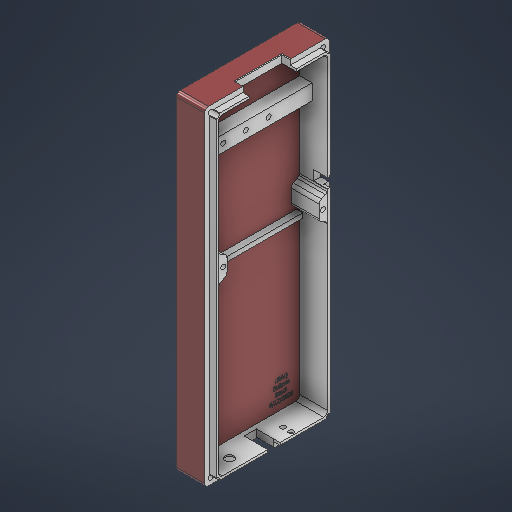
# Autodesk Inventor part: cDAQ_Bottom_Box3
Saved by Autodesk Inventor 2027 (Build 310192000, 192)
## iProperties
Created: 2026-05-08
Part Number: cDAQ_Bottom_Box3
Material: Generic
Document SubType Name: Modeling
Designer: giese
Density: 1 g/cm^3
Appearance: Default
Author: giese
Autodesk Inventor part; units mm, degrees
(part 1 of 2)
ref_plane "YZ Plane" through (0, 0, 0) normal (1, 0, 0) x (0, 1, 0)
ref_plane "XZ Plane" through (0, 0, 0) normal (0, 1, 0) x (-1, 0, 0)
ref_plane "XY Plane" through (0, 0, 0) normal (0, 0, 1) x (1, 0, 0)
sketch "Sketch1" plane through (0, 0, 0) normal (1, 0, 0) x (0, 1, 0)
  line L0 (37.5698, 53.1667) -> (-230.1462, 53.1667)
  line L1 (-230.1462, 53.1667) -> (-230.1462, -48.4333)
  line L2 (-230.1462, -48.4333) -> (37.5698, -48.4333)
  line L3 (37.5698, -48.4333) -> (37.5698, 53.1667)
  point P0 (0, 0)
  dimension "d0" = 101.6
  dimension "d1" = 267.716
  constraints: 8 end point, 2 parallel, 1 horizontal, 1 perpendicular
  measures "d0" distance of L2.end L0.start
  measures "d1" distance of L1.end L2.end
extrude "Extrusion1" add sketch "Sketch1" along normal blind 22.86
sketch "Sketch2" plane through (22.86, 0, 0) normal (1, 0, 0) x (0, 0, -1)
  line L0 (42.0833, 31.2198) -> (-46.8167, 31.2198)
  line L1 (-46.8167, 31.2198) -> (-46.8167, -223.7962)
  line L2 (-46.8167, -223.7962) -> (42.0833, -223.7962)
  line L3 (42.0833, -223.7962) -> (42.0833, 31.2198)
  line L4 (48.4333, 37.5698) -> (-53.1667, 37.5698) projected
  line L5 (-53.1667, 37.5698) -> (-53.1667, -230.1462) projected
  line L6 (-53.1667, -230.1462) -> (48.4333, -230.1462) projected
  point P0 (0, 0)
  dimension "d4" = 255.016
  dimension "d5" = 88.9
  dimension "d8" = 6.35
  dimension "d21" = 6.35
  dimension "d690" = 6.35
  constraints: 8 end point, 2 parallel, 1 horizontal, 1 perpendicular
  measures "d4" distance of L2.end L0.start
  measures "d5" distance of L0.start L0.end
  measures "d8" distance between parallel lines of L0 L4
  measures "d21" distance between parallel lines of L5 L1
  measures "d690" distance between parallel lines of L6 L2
extrude "Extrusion2" cut sketch "Sketch2" against normal blind 17.78
sketch "Sketch3" plane through (0, 0, 0) normal (-1, 0, 0) x (0, 0, 1)
  circle A0 centre (-6.6909, -2.0542) radius 2
  circle A1 centre (11.8079, -2.0542) radius 2
  circle A2 centre (30.3067, -2.0542) radius 2
  line L0 (-48.4333, -230.1462) -> (-48.4333, 37.5698) projected
  line L1 (-48.4333, 37.5698) -> (53.1667, 37.5698) projected
  line L2 (53.1667, 37.5698) -> (53.1667, -230.1462) projected
  line L3 (46.8167, 31.2198) -> (-42.0833, 31.2198) projected
  point P0 (0, 0)
  point P1 (-0.896, -23.7433)
  point P2 (-45.1848, 27.0137)
  dimension "d9" = 18.4988
  dimension "d10" = 4
  dimension "d11" = 4
  dimension "d12" = 18.4988
  dimension "d13" = 36.9976
  dimension "d18" = 22.86
  dimension "d22" = 4
  dimension "d58" = 39.624
  constraints: 3 centre point
  measures "d9" distance of A0.centre A1.centre
  measures "d10" diameter of A1
  measures "d11" diameter of A2
  measures "d12" distance of A1.centre A2.centre
  measures "d13" distance of A0.centre A2.centre
  measures "d18" distance from line of L2 A2.centre
  measures "d22" diameter of A0
  measures "d58" distance from line of L1 A2.centre
extrude "Extrusion3" cut sketch "Sketch3" against normal blind 5.08
sketch "Sketch5" plane through (0, -230.1462, -48.4333) normal (0, 0, -1) x (-1, 0, 0)
  line L0 (-27.2034, 165.862) -> (-16.51, 165.862)
  line L1 (-16.51, 165.862) -> (-16.51, 173.862)
  line L2 (-16.51, 173.862) -> (-27.2034, 173.862)
  line L3 (-27.2034, 173.862) -> (-27.2034, 165.862)
  line L4 (0, 267.716) -> (-22.86, 267.716) projected
  line L5 (0, 0) -> (0, 267.716) projected
  line L6 (-22.86, 0) -> (-22.86, 267.716) projected
  point P0 (0, 230.1462)
  point P1 (-21.8567, 173.862)
  point P2 (-21.8567, 165.862)
  dimension "d28" = 10.6934
  dimension "d30" = 8
  dimension "d31" = 16.51
  dimension "d34" = 101.854
  dimension "d215" = 4.3434
  constraints: 8 end point, 2 midpoint, 2 parallel, 1 horizontal, 1 perpendicular
  measures "d28" distance between parallel lines of L1 L3
  measures "d30" distance of point (-21.857, 173.862) point (-21.857, 165.862)
  measures "d31" distance between parallel lines of L5 L1
  measures "d34" distance between parallel lines of L4 L0
  measures "d215" distance between parallel lines of L6 L3
extrude "Extrusion4" cut sketch "Sketch5" against normal blind 24.13
sketch "Sketch6" plane through (0, -230.1462, -48.4333) normal (0, -1, 0) x (1, 0, 0)
  line L0 (24.08, 55.136) -> (16.08, 55.136)
  line L1 (16.08, 45.136) -> (24.08, 45.136)
  line L2 (0, 101.6) -> (0, 0) projected
  line L3 (28.36, 53.1359) -> (28.36, 47.136)
  line L4 (24.08, 55.136) -> (28.36, 53.1359)
  line L5 (28.36, 47.136) -> (24.08, 45.136)
  line L6 (0, 0) -> (22.86, 0) projected
  line L7 (22.86, 95.25) -> (22.86, 6.35) projected
  line L8 (22.86, 41.9134) -> (22.86, 37.4697)
  line L9 (16.08, 55.136) -> (8.636, 55.136)
  line L10 (8.636, 55.136) -> (8.636, 45.136)
  line L11 (8.636, 45.136) -> (21.16, 45.136)
  point P0 (0, 48.4333)
  point P1 (20.08, 55.136)
  point P2 (20.08, 45.136)
  point P3 (16.08, 50.136)
  dimension "d39" = 6
  dimension "d48" = 55.136
  dimension "d221" = 0
  dimension "d223" = 2
  dimension "d224" = 2
  dimension "d225" = 5.5
  dimension "d227" = 4.28
  dimension "d672" = 8.636
  constraints: 18 end point, 2 horizontal, 2 midpoint, 2 parallel, 2 point on line, 1 perpendicular, 1 vertical
  measures "d39" distance of L3.start L3.end
  measures "d48" distance between parallel lines of L6 L0
  measures "d221" horizontal distance of L0.start L1.end
  measures "d223" vertical distance of L3.end L1.end
  measures "d224" vertical distance of L0.start L3.start
  measures "d225" distance between parallel lines of L3 L7
  measures "d227" distance from line of L1.end L3
  measures "d672" distance between parallel lines of L2 L10
extrude "Extrusion5" cut sketch "Sketch6" against normal blind 6.35
sketch "Sketch7" plane through (0, 37.5698, 53.1667) normal (0, 1, 0) x (1, 0, 0)
  line L0 (31.0134, 69.85) -> (16.002, 69.85)
  line L1 (16.002, 69.85) -> (16.002, 31.75)
  line L2 (16.002, 31.75) -> (31.0134, 31.75)
  line L3 (31.0134, 31.75) -> (31.0134, 69.85)
  line L4 (0, 0) -> (22.86, 0) projected
  line L5 (0, 101.6) -> (0, 0) projected
  line L6 (22.86, 101.6) -> (22.86, 0) projected
  point P0 (0, 53.1667)
  point P1 (22.86, 69.85)
  point P2 (22.86, 31.75)
  dimension "d51" = 38.1
  dimension "d52" = 31.75
  dimension "d55" = 16.002
  dimension "d56" = 15.0114
  dimension "d57" = 8.1534
  constraints: 8 end point, 2 parallel, 1 horizontal, 1 perpendicular
  measures "d51" distance of L2.end L0.start
  measures "d52" distance between parallel lines of L4 L2
  measures "d55" distance between parallel lines of L5 L1
  measures "d56" distance between parallel lines of L3 L1
  measures "d57" distance between parallel lines of L6 L3
extrude "Extrusion6" cut sketch "Sketch7" against normal blind 7.62
fillet "Fillet1" radius 3.175 4 edges at (11.43, 37.5698, -48.4333) (11.43, 37.5698, 53.1667) (11.43, -230.1462, -48.4333) (11.43, -230.1462, 53.1667)
sketch "Sketch8" plane through (0, 0, 0) normal (-1, 0, 0) x (0, 0, 1)
  line L0 (-8.4625, -5.5848) -> (-4.9319, -5.5848)
  line L1 (-8.4625, 1.4764) -> (-4.9319, 1.4764)
  line L2 (-8.4625, -5.5848) -> (-10.5009, -2.0542)
  line L3 (-8.4625, 1.4764) -> (-10.5009, -2.0542)
  line L4 (-4.9319, -5.5848) -> (-2.8936, -2.0542)
  line L5 (-4.9319, 1.4764) -> (-2.8936, -2.0542)
  circle A0 centre (-6.6909, -2.0542) radius 2 projected
  line L6 (10.0363, -5.5848) -> (13.5669, -5.5848)
  line L7 (10.0363, 1.4764) -> (13.5669, 1.4764)
  line L8 (10.0363, -5.5848) -> (7.9979, -2.0542)
  line L9 (10.0363, 1.4764) -> (7.9979, -2.0542)
  line L10 (13.5669, -5.5848) -> (15.6053, -2.0542)
  line L11 (13.5669, 1.4764) -> (15.6053, -2.0542)
  circle A1 centre (11.8079, -2.0542) radius 2 projected
  line L12 (28.5351, -5.5848) -> (26.4967, -2.0542)
  line L13 (28.5351, 1.4764) -> (26.4967, -2.0542)
  line L14 (28.5351, -5.5848) -> (32.0657, -5.5848)
  line L15 (28.5351, 1.4764) -> (32.0657, 1.4764)
  line L16 (32.0657, -5.5848) -> (34.1041, -2.0542)
  line L17 (32.0657, 1.4764) -> (34.1041, -2.0542)
  circle A2 centre (30.3067, -2.0542) radius 2 projected
  point P0 (-6.6972, -5.5848)
  point P1 (11.8016, -5.5848)
  point P2 (30.3004, -5.5848)
  point P3 (-10.5009, -2.0542)
  point P4 (-2.8936, -2.0542)
  point P5 (15.6053, -2.0542)
  point P6 (7.9979, -2.0542)
  point P7 (34.1041, -2.0542)
  point P8 (26.4967, -2.0542)
  dimension "d60" = 7.0612
  dimension "d61" = 120
  dimension "d62" = 120
  dimension "d63" = 120
  dimension "d64" = 120
  dimension "d65" = 3.5306
  dimension "d66" = 3.5306
  dimension "d67" = 3.5306
  dimension "d68" = 3.5306
  dimension "d69" = 3.5306
  dimension "d70" = 3.5306
  dimension "d71" = 0
  dimension "d72" = 7.6074
  dimension "d73" = 3.81
  dimension "d74" = 0
  dimension "d75" = 7.0612
  dimension "d76" = 120
  dimension "d77" = 120
  dimension "d78" = 120
  dimension "d79" = 120
  dimension "d80" = 3.5306
  dimension "d81" = 3.5306
  dimension "d82" = 3.5306
  dimension "d83" = 3.5306
  dimension "d84" = 3.5306
  dimension "d85" = 3.5306
  dimension "d86" = 0
  dimension "d87" = 7.6074
  dimension "d91" = 0
  dimension "d92" = 3.81
  dimension "d93" = 7.0612
  dimension "d94" = 120
  dimension "d95" = 120
  dimension "d96" = 120
  dimension "d97" = 120
  dimension "d98" = 3.5306
  dimension "d99" = 3.5306
  dimension "d100" = 3.5306
  dimension "d101" = 3.5306
  dimension "d102" = 3.5306
  dimension "d103" = 3.5306
  dimension "d104" = 0
  dimension "d105" = 7.6074
  dimension "d108" = 0
  dimension "d109" = 3.81
  constraints: 36 end point, 6 horizontal, 3 midpoint
  measures "d60" distance from line of point (-6.697, -5.585) L1
  measures "d61" angle of L0 L2
  measures "d62" angle of L1 L3
  measures "d63" angle of L4 L0
  measures "d64" angle of L5 L1
  measures "d65" distance of L0.start L0.end
  measures "d66" distance of L1.start L1.end
  measures "d67" vertical distance of L1.start L3.end
  measures "d68" vertical distance of L0.start L2.end
  measures "d69" vertical distance of L1.end L5.end
  measures "d70" vertical distance of L0.end L4.end
  measures "d71" horizontal distance of L0.start L1.start
  measures "d72" distance of L4.end L2.end
  measures "d73" distance of A0.centre L2.end
  measures "d74" vertical distance of A0.centre L4.end
  measures "d75" distance from line of point (11.802, -5.585) L7
  measures "d76" angle of L6 L8
  measures "d77" angle of L7 L9
  measures "d78" angle of L10 L6
  measures "d79" angle of L11 L7
  measures "d80" distance of L8.start L6.end
  measures "d81" distance of L9.start L7.end
  measures "d82" vertical distance of L9.start L9.end
  measures "d83" vertical distance of L8.start L8.end
  measures "d84" vertical distance of L7.end L11.end
  measures "d85" vertical distance of L6.end L10.end
  measures "d86" horizontal distance of L8.start L9.start
  measures "d87" distance of L10.end L8.end
  measures "d91" vertical distance of A1.centre L8.end
  measures "d92" distance of A1.centre L8.end
  measures "d93" distance from line of point (30.3, -5.585) L15
  measures "d94" angle of L14 L12
  measures "d95" angle of L15 L13
  measures "d96" angle of L16 L14
  measures "d97" angle of L17 L15
  measures "d98" distance of L12.start L16.start
  measures "d99" distance of L15.start L15.end
  measures "d100" vertical distance of L15.start L13.end
  measures "d101" vertical distance of L12.start L12.end
  measures "d102" vertical distance of L15.end L17.end
  measures "d103" vertical distance of L16.start L16.end
  measures "d104" horizontal distance of L12.start L15.start
  measures "d105" distance of L16.end L12.end
  measures "d108" vertical distance of A2.centre L12.end
  measures "d109" distance of A2.centre L12.end
extrude "Extrusion7" cut sketch "Sketch8" against normal blind 4 contours L2 L3 L1 L5 L4 L0 | A0 | L8 L9 L7 L11 L10 L6 | A1 | L12 L13 L15 L17 L16 L14 | A2
sketch "Sketch9" plane through (5.08, 0, 0) normal (1, 0, 0) x (0, 0, -1)
  arc A0 (24.8089, -180.8044) -> (19.3527, -180.8044) centre (22.0808, -178.3302) ccw
  line L0 (45.2583, 37.5698) -> (16.6833, 37.5698) projected
  line L1 (42.0833, 31.2198) -> (42.0833, -223.7962) projected
  arc A1 (20.1758, -185.9502) -> (23.9858, -185.9502) centre (22.0808, -185.9502) ccw
  line L2 (23.9858, -185.9502) -> (23.9858, -182.9374)
  line L3 (20.1758, -185.9502) -> (20.1758, -182.9374)
  arc A2 (24.8089, -180.8044) -> (23.9858, -182.9374) centre (27.1608, -182.9374) ccw
  arc A3 (20.1758, -182.9374) -> (19.3527, -180.8044) centre (17.0008, -182.9374) ccw
  arc A4 (-25.9911, -180.8044) -> (-31.4473, -180.8045) centre (-28.7192, -178.3302) ccw
  arc A5 (-30.6242, -185.9366) -> (-26.8142, -185.9502) centre (-28.7192, -185.9502) ccw
  line L4 (-26.8142, -185.9502) -> (-26.8142, -182.9374)
  line L5 (-30.6242, -185.9366) -> (-30.6242, -182.9374)
  arc A6 (-25.9911, -180.8044) -> (-26.8142, -182.9374) centre (-23.6392, -182.9374) ccw
  arc A7 (-30.6242, -182.9374) -> (-31.4473, -180.8045) centre (-33.7992, -182.9374) ccw
  line L6 (-21.4167, 37.5698) -> (-49.9917, 37.5698) projected
  line L7 (-46.8167, -223.7962) -> (-46.8167, 31.2198) projected
  point P0 (0, 0)
  point P1 (23.9858, -181.4823)
  point P2 (20.1758, -181.4823)
  point P3 (-26.8142, -181.4823)
  point P4 (-30.6242, -181.4823)
  dimension "d112" = 215.9
  dimension "d114" = 7.366
  dimension "d116" = 3.81
  dimension "d117" = 223.52
  dimension "d118" = 3.175
  dimension "d119" = 7.366
  dimension "d120" = 3.81
  dimension "d121" = 3.175
  dimension "d122" = 215.9
  dimension "d123" = 223.52
  dimension "d125" = 0
  dimension "d128" = 50.8
  dimension "d129" = 20.0025
  dimension "d130" = 0
  constraints: 20 point on circle, 8 centre point, 8 end point, 8 tangent, 4 point on line, 2 equal radius, 2 parallel, 2 vertical
  measures "d112" distance from line of L0 A0.centre
  measures "d114" diameter of A0
  measures "d116" diameter of A1
  measures "d117" distance from line of L0 A1.centre
  measures "d118" radius of A2
  measures "d119" diameter of A4
  measures "d120" diameter of A5
  measures "d121" radius of A6
  measures "d122" distance from line of A4.centre L6
  measures "d123" distance from line of L6 A5.centre
  measures "d125" horizontal distance of A5.centre A4.centre
  measures "d128" distance of A5.centre A1.centre
  measures "d129" distance from line of L1 A0.centre
  measures "d130" horizontal distance of A0.centre A1.centre
extrude "Extrusion8" [suppressed]
sketch "Sketch10" plane through (22.86, 0, 0) normal (1, 0, 0) x (0, 0, -1)
  line L0 (-46.8167, 31.2198) -> (42.0833, 31.2198) projected
  line L1 (-46.8167, 31.2198) -> (42.0833, 31.2198)
  line L2 (42.0833, 33.2264) -> (-46.8167, 33.2264)
  line L3 (-46.8167, 33.2264) -> (-48.8233, 33.2264)
  line L4 (-48.8233, 33.2264) -> (-48.8233, -225.8028)
  line L5 (-48.8233, -225.8028) -> (44.0899, -225.8028)
  line L6 (44.0899, -225.8028) -> (44.0899, 33.2264)
  line L7 (44.0899, 33.2264) -> (41.9392, 33.2264)
  line L8 (42.0833, 31.2198) -> (42.0833, -223.7962) projected
  line L9 (-46.8167, -223.7962) -> (-46.8167, 31.2198) projected
  line L10 (42.0833, -223.7962) -> (-46.8167, -223.7962) projected
  line L11 (45.2583, 37.5698) -> (16.6833, 37.5698) projected
  dimension "d202" = 2.0066
  dimension "d203" = 2.0066
  dimension "d204" = 2.0066
  dimension "d205" = 2.0066
  dimension "d208" = 4.3434
  constraints: 14 end point, 3 perpendicular, 3 point on line, 1 collinear, 1 horizontal
  measures "d202" distance between parallel lines of L0 L2
  measures "d203" distance between parallel lines of L6 L8
  measures "d204" distance between parallel lines of L4 L9
  measures "d205" distance between parallel lines of L5 L10
  measures "d208" distance between parallel lines of L11 L2
extrude "Extrusion9" add sketch "Sketch10" along normal blind 5
fillet "Fillet2" radius 3.175 8 edges at (16.47, 31.2198, -42.0833) (16.47, 31.2198, 46.8167) (16.47, -223.7962, 46.8167) (16.47, -223.7962, -42.0833) (25.36, 33.2264, -44.0899) (25.36, 33.2264, 48.8233) (25.36, -225.8028, -44.0899) (25.36, -225.8028, 48.8233)
sketch "Sketch13" plane through (27.86, 0, 0) normal (1, 0, 0) x (0, 0, -1)
  arc A0 (44.0833, 30.0448) -> (40.9083, 33.2198) centre (40.9083, 30.0448) ccw projected
  arc A1 (-45.6417, 33.2198) -> (-48.8167, 30.0448) centre (-45.6417, 30.0448) ccw projected
  arc A2 (40.9083, -212.0802) -> (44.0833, -208.9052) centre (40.9083, -208.9052) ccw projected
  arc A3 (-48.8167, -208.9052) -> (-45.6417, -212.0802) centre (-45.6417, -208.9052) ccw projected
  line L0 (-21.4167, 37.5698) -> (-49.9917, 37.5698) projected
  line L1 (-53.1667, 34.3948) -> (-53.1667, -226.9712) projected
  line L2 (-49.9917, -230.1462) -> (45.2583, -230.1462) projected
  arc A4 (-48.8167, -208.9052) -> (-45.6417, -212.0802) centre (-45.6417, -208.9052) ccw projected
  circle A5 centre (-48.0867, -225.0662) radius 1.9939
  circle A6 centre (43.3533, -225.0662) radius 1.9939
  line L3 (48.4333, -226.9712) -> (48.4333, 34.3948) projected
  circle A7 centre (43.3533, 32.4898) radius 1.9939
  line L4 (45.2583, 37.5698) -> (16.6833, 37.5698) projected
  circle A8 centre (-48.0867, 32.4898) radius 1.9939
  arc A9 (41.4904, -28.6131) -> (38.3154, -25.4381) centre (38.3154, -28.6131) ccw
  circle A10 centre (38.2733, -76.7302) radius 1.9939
  circle A11 centre (-43.0067, -76.7302) radius 1.9939
  point P0 (0, 0)
  point P1 (-47.8868, 32.2898)
  point P2 (-47.8868, -211.1503)
  point P3 (-47.8868, -211.1503)
  point P4 (45.8404, -24.2631)
  point P5 (42.6654, -21.0881)
  dimension "d389" = 3.5306
  dimension "d178" = 5.08
  dimension "d179" = 5.08
  dimension "d180" = 3.9878
  dimension "d181" = 5.08
  dimension "d182" = 5.08
  dimension "d183" = 3.9878
  dimension "d184" = 3.9878
  dimension "d185" = 5.08
  dimension "d186" = 5.08
  dimension "d187" = 3.9878
  dimension "d188" = 5.08
  dimension "d189" = 5.08
  dimension "d326" = 3.9878
  dimension "d327" = 10.16
  dimension "d328" = 114.3
  dimension "d329" = 3.9878
  dimension "d330" = 10.16
  dimension "d331" = 114.3
  constraints: 7 centre point, 5 point on circle
  measures "d178" distance from line of L1 A5.centre
  measures "d179" distance from line of L2 A5.centre
  measures "d180" diameter of A5
  measures "d181" distance from line of L2 A6.centre
  measures "d182" distance from line of L3 A6.centre
  measures "d183" diameter of A6
  measures "d184" diameter of A7
  measures "d185" distance from line of L3 A7.centre
  measures "d186" distance from line of L4 A7.centre
  measures "d187" diameter of A8
  measures "d188" distance from line of L0 A8.centre
  measures "d189" distance from line of L1 A8.centre
  measures "d326" diameter of A10
  measures "d327" distance from line of L3 A10.centre
  measures "d328" distance from line of A10.centre L4
  measures "d329" diameter of A11
  measures "d330" distance from line of L1 A11.centre
  measures "d331" distance from line of L0 A11.centre
extrude "Extrusion11" cut sketch "Sketch13" against normal blind 25.4
sketch "Sketch14" plane through (5.08, 0, 0) normal (1, 0, 0) x (0, 0, -1)
  line L0 (17.4136, -199.8901) -> (36.6303, -199.8901) construction
  line L1 (36.6303, -199.8901) -> (36.6303, -208.6828) construction
  line L2 (36.6303, -208.6828) -> (17.4136, -208.6828) construction
  line L3 (17.4136, -208.6828) -> (17.4136, -199.8901) construction
  spline S0 degree 2 poles (23.081, -203.0542) (22.8439, -203.0542) (22.4512, -202.9085) (22.3104, -202.7603) knots 0 0 0 1 2 2 2
  spline S1 degree 2 poles (22.3104, -202.7603) (22.1696, -202.6146) (22.014, -202.165) (22.014, -201.8637) knots 0 0 0 1 2 2 2
  spline S2 degree 2 poles (22.014, -201.8637) (22.014, -201.5624) (22.1745, -201.1227) (22.3104, -200.9745) knots 0 0 0 1 2 2 2
  spline S3 degree 2 poles (22.3104, -200.9745) (22.4463, -200.8238) (22.8489, -200.6633) (23.081, -200.6633) knots 0 0 0 1 2 2 2
  spline S4 degree 2 poles (23.081, -200.6633) (23.2688, -200.6633) (23.6195, -200.7695) (23.7554, -200.8386) knots 0 0 0 1 2 2 2
  line L4 (23.7554, -200.8386) -> (23.7554, -201.2709)
  line L5 (23.7554, -201.2709) -> (23.7331, -201.2709)
  spline S5 degree 2 poles (23.7331, -201.2709) (23.6911, -201.2363) (23.5627, -201.1474) (23.4713, -201.1005) knots 0 0 0 1 2 2 2
  spline S6 degree 2 poles (23.4713, -201.1005) (23.3898, -201.0609) (23.1724, -200.9992) (23.0736, -200.9992) knots 0 0 0 1 2 2 2
  spline S7 degree 2 poles (23.0736, -200.9992) (22.7748, -200.9992) (22.4117, -201.4512) (22.4117, -201.8637) knots 0 0 0 1 2 2 2
  spline S8 degree 2 poles (22.4117, -201.8637) (22.4117, -202.2663) (22.7624, -202.7183) (23.0736, -202.7183) knots 0 0 0 1 2 2 2
  spline S9 degree 2 poles (23.0736, -202.7183) (23.2614, -202.7183) (23.6022, -202.5627) (23.7331, -202.4417) knots 0 0 0 1 2 2 2
  line L6 (23.7331, -202.4417) -> (23.7554, -202.4417)
  line L7 (23.7554, -202.4417) -> (23.7554, -202.8739)
  spline S10 degree 2 poles (23.7554, -202.8739) (23.6985, -202.9011) (23.5256, -202.9777) (23.4565, -202.995) knots 0 0 0 1 2 2 2
  spline S11 degree 2 poles (23.4565, -202.995) (23.3577, -203.0246) (23.2021, -203.0542) (23.081, -203.0542) knots 0 0 0 1 2 2 2
  spline S12 degree 2 poles (26.5391, -201.4808) (26.5391, -201.8983) (26.2007, -202.5701) (25.9166, -202.7578) knots 0 0 0 1 2 2 2
  spline S13 degree 2 poles (25.9166, -202.7578) (25.6844, -202.9036) (25.2077, -203.0024) (24.8372, -203.0024) knots 0 0 0 1 2 2 2
  line L8 (24.8372, -203.0024) -> (24.1357, -203.0024)
  line L9 (24.1357, -203.0024) -> (24.1357, -199.9544)
  line L10 (24.1357, -199.9544) -> (24.8298, -199.9544)
  spline S14 degree 2 poles (24.8298, -199.9544) (25.2596, -199.9544) (25.7487, -200.0828) (25.9216, -200.1964) knots 0 0 0 1 2 2 2
  spline S15 degree 2 poles (25.9216, -200.1964) (26.2155, -200.3916) (26.5391, -201.0362) (26.5391, -201.4808) knots 0 0 0 1 2 2 2
  spline S16 degree 2 poles (26.1167, -201.4759) (26.1167, -201.1252) (25.8845, -200.6287) (25.6548, -200.4879) knots 0 0 0 1 2 2 2
  spline S17 degree 2 poles (25.6548, -200.4879) (25.4918, -200.3916) (25.1237, -200.3051) (24.8496, -200.3051) knots 0 0 0 1 2 2 2
  line L11 (24.8496, -200.3051) -> (24.5408, -200.3051)
  line L12 (24.5408, -200.3051) -> (24.5408, -202.6516)
  line L13 (24.5408, -202.6516) -> (24.8496, -202.6516)
  spline S18 degree 2 poles (24.8496, -202.6516) (25.1188, -202.6516) (25.5264, -202.5652) (25.6919, -202.4491) knots 0 0 0 1 2 2 2
  spline S19 degree 2 poles (25.6919, -202.4491) (25.9043, -202.3058) (26.1167, -201.8316) (26.1167, -201.4759) knots 0 0 0 1 2 2 2
  line L14 (26.6502, -203.0024) -> (27.6777, -199.9544)
  line L15 (27.6777, -199.9544) -> (28.1767, -199.9544)
  line L16 (28.1767, -199.9544) -> (29.2042, -203.0024)
  line L17 (29.2042, -203.0024) -> (28.7769, -203.0024)
  line L18 (28.7769, -203.0024) -> (28.5003, -202.1502)
  line L19 (28.5003, -202.1502) -> (27.3369, -202.1502)
  line L20 (27.3369, -202.1502) -> (27.0602, -203.0024)
  line L21 (27.0602, -203.0024) -> (26.6502, -203.0024)
  line L22 (28.3891, -201.8044) -> (27.9173, -200.3693)
  line L23 (27.9173, -200.3693) -> (27.448, -201.8044)
  line L24 (27.448, -201.8044) -> (28.3891, -201.8044)
  spline S20 degree 2 poles (32.025, -203.7483) (31.9138, -203.7755) (31.6718, -203.8051) (31.5507, -203.8051) knots 0 0 0 1 2 2 2
  spline S21 degree 2 poles (31.5507, -203.8051) (31.2074, -203.8051) (30.7801, -203.4223) (30.7603, -203.0666) knots 0 0 0 1 2 2 2
  spline S22 degree 2 poles (30.7603, -203.0666) (30.7332, -203.0666) (30.6862, -203.0666) (30.6665, -203.0666) knots 0 0 0 1 2 2 2
  spline S23 degree 2 poles (30.6665, -203.0666) (30.3577, -203.0666) (29.8612, -202.8566) (29.6834, -202.6516) knots 0 0 0 1 2 2 2
  spline S24 degree 2 poles (29.6834, -202.6516) (29.508, -202.4491) (29.3203, -201.8563) (29.3203, -201.4808) knots 0 0 0 1 2 2 2
  spline S25 degree 2 poles (29.3203, -201.4808) (29.3203, -201.0955) (29.5105, -200.5126) (29.6859, -200.3051) knots 0 0 0 1 2 2 2
  spline S26 degree 2 poles (29.6859, -200.3051) (29.8637, -200.1001) (30.3602, -199.8901) (30.6665, -199.8901) knots 0 0 0 1 2 2 2
  spline S27 degree 2 poles (30.6665, -199.8901) (30.9777, -199.8901) (31.4766, -200.1075) (31.6495, -200.3051) knots 0 0 0 1 2 2 2
  spline S28 degree 2 poles (31.6495, -200.3051) (31.8224, -200.5052) (32.0151, -201.1005) (32.0151, -201.4808) knots 0 0 0 1 2 2 2
  spline S29 degree 2 poles (32.0151, -201.4808) (32.0151, -202.0736) (31.5532, -202.8443) (31.1506, -202.9801) knots 0 0 0 1 2 2 2
  spline S30 degree 2 poles (31.1506, -202.9801) (31.1605, -203.0938) (31.2197, -203.2765) (31.2667, -203.3284) knots 0 0 0 1 2 2 2
  spline S31 degree 2 poles (31.2667, -203.3284) (31.3235, -203.3926) (31.4791, -203.4519) (31.6174, -203.4519) knots 0 0 0 1 2 2 2
  spline S32 degree 2 poles (31.6174, -203.4519) (31.6989, -203.4519) (31.9212, -203.4) (31.9706, -203.3803) knots 0 0 0 1 2 2 2
  line L25 (31.9706, -203.3803) -> (32.025, -203.3803)
  line L26 (32.025, -203.3803) -> (32.025, -203.7483)
  spline S33 degree 2 poles (31.5927, -201.4808) (31.5927, -201.177) (31.4618, -200.7102) (31.3433, -200.5571) knots 0 0 0 1 2 2 2
  spline S34 degree 2 poles (31.3433, -200.5571) (31.2222, -200.399) (30.8814, -200.2409) (30.6689, -200.2409) knots 0 0 0 1 2 2 2
  spline S35 degree 2 poles (30.6689, -200.2409) (30.4491, -200.2409) (30.1181, -200.394) (29.9922, -200.5571) knots 0 0 0 1 2 2 2
  spline S36 degree 2 poles (29.9922, -200.5571) (29.8711, -200.7127) (29.7427, -201.1844) (29.7427, -201.4808) knots 0 0 0 1 2 2 2
  spline S37 degree 2 poles (29.7427, -201.4808) (29.7427, -202.0811) (30.2466, -202.7208) (30.6689, -202.7208) knots 0 0 0 1 2 2 2
  spline S38 degree 2 poles (30.6689, -202.7208) (31.0913, -202.7208) (31.5927, -202.0811) (31.5927, -201.4808) knots 0 0 0 1 2 2 2
  spline S39 degree 2 poles (22.7254, -207.0847) (22.7254, -207.3119) (22.5525, -207.6602) (22.4092, -207.7738) knots 0 0 0 1 2 2 2
  spline S40 degree 2 poles (22.4092, -207.7738) (22.2363, -207.9072) (21.8436, -208.0208) (21.5323, -208.0208) knots 0 0 0 1 2 2 2
  line L27 (21.5323, -208.0208) -> (20.658, -208.0208)
  line L28 (20.658, -208.0208) -> (20.658, -204.9728)
  line L29 (20.658, -204.9728) -> (21.4657, -204.9728)
  spline S41 degree 2 poles (21.4657, -204.9728) (21.7917, -204.9728) (22.1177, -205.0148) (22.2659, -205.0963) knots 0 0 0 1 2 2 2
  spline S42 degree 2 poles (22.2659, -205.0963) (22.4314, -205.1828) (22.5821, -205.4668) (22.5821, -205.6595) knots 0 0 0 1 2 2 2
  spline S43 degree 2 poles (22.5821, -205.6595) (22.5821, -205.8744) (22.3549, -206.2152) (22.1548, -206.3116) knots 0 0 0 1 2 2 2
  line L30 (22.1548, -206.3116) -> (22.1548, -206.3264)
  spline S44 degree 2 poles (22.1548, -206.3264) (22.4265, -206.4005) (22.7254, -206.7932) (22.7254, -207.0847) knots 0 0 0 1 2 2 2
  spline S45 degree 2 poles (22.303, -207.102) (22.303, -206.9291) (22.2042, -206.7068) (22.056, -206.6277) knots 0 0 0 1 2 2 2
  spline S46 degree 2 poles (22.056, -206.6277) (21.9597, -206.5783) (21.7324, -206.5487) (21.5225, -206.5487) knots 0 0 0 1 2 2 2
  line L31 (21.5225, -206.5487) -> (21.063, -206.5487)
  line L32 (21.063, -206.5487) -> (21.063, -207.675)
  line L33 (21.063, -207.675) -> (21.3916, -207.675)
  spline S47 degree 2 poles (21.3916, -207.675) (21.6583, -207.675) (21.9646, -207.6256) (22.0832, -207.5466) knots 0 0 0 1 2 2 2
  spline S48 degree 2 poles (22.0832, -207.5466) (22.1968, -207.4651) (22.303, -207.2625) (22.303, -207.102) knots 0 0 0 1 2 2 2
  spline S49 degree 2 poles (22.1597, -205.7163) (22.1597, -205.6076) (22.0856, -205.4446) (22.0041, -205.3977) knots 0 0 0 1 2 2 2
  spline S50 degree 2 poles (22.0041, -205.3977) (21.9053, -205.3433) (21.6657, -205.3186) (21.4508, -205.3186) knots 0 0 0 1 2 2 2
  line L34 (21.4508, -205.3186) -> (21.063, -205.3186)
  line L35 (21.063, -205.3186) -> (21.063, -206.2103)
  line L36 (21.063, -206.2103) -> (21.5225, -206.2103)
  spline S51 degree 2 poles (21.5225, -206.2103) (21.7127, -206.2103) (21.893, -206.1708) (21.9893, -206.109) knots 0 0 0 1 2 2 2
  spline S52 degree 2 poles (21.9893, -206.109) (22.0832, -206.0497) (22.1597, -205.8596) (22.1597, -205.7163) knots 0 0 0 1 2 2 2
  spline S53 degree 2 poles (24.978, -206.8772) (24.978, -207.4552) (24.4223, -208.085) (23.9579, -208.085) knots 0 0 0 1 2 2 2
  spline S54 degree 2 poles (23.9579, -208.085) (23.4812, -208.085) (22.9353, -207.4354) (22.9353, -206.8772) knots 0 0 0 1 2 2 2
  spline S55 degree 2 poles (22.9353, -206.8772) (22.9353, -206.3042) (23.4985, -205.6694) (23.9579, -205.6694) knots 0 0 0 1 2 2 2
  spline S56 degree 2 poles (23.9579, -205.6694) (24.4223, -205.6694) (24.978, -206.3017) (24.978, -206.8772) knots 0 0 0 1 2 2 2
  spline S57 degree 2 poles (24.5803, -206.8772) (24.5803, -206.4326) (24.2568, -206.0003) (23.9579, -206.0003) knots 0 0 0 1 2 2 2
  spline S58 degree 2 poles (23.9579, -206.0003) (23.659, -206.0003) (23.333, -206.4326) (23.333, -206.8772) knots 0 0 0 1 2 2 2
  spline S59 degree 2 poles (23.333, -206.8772) (23.333, -207.3095) (23.659, -207.7541) (23.9579, -207.7541) knots 0 0 0 1 2 2 2
  spline S60 degree 2 poles (23.9579, -207.7541) (24.2543, -207.7541) (24.5803, -207.3169) (24.5803, -206.8772) knots 0 0 0 1 2 2 2
  spline S61 degree 2 poles (26.0648, -208.0653) (25.7511, -208.0653) (25.3979, -207.7071) (25.3979, -207.3193) knots 0 0 0 1 2 2 2
  line L37 (25.3979, -207.3193) -> (25.3979, -206.0522)
  line L38 (25.3979, -206.0522) -> (25.1386, -206.0522)
  line L39 (25.1386, -206.0522) -> (25.1386, -205.7336)
  line L40 (25.1386, -205.7336) -> (25.3979, -205.7336)
  line L41 (25.3979, -205.7336) -> (25.3979, -205.0766)
  line L42 (25.3979, -205.0766) -> (25.7832, -205.0766)
  line L43 (25.7832, -205.0766) -> (25.7832, -205.7336)
  line L44 (25.7832, -205.7336) -> (26.4921, -205.7336)
  line L45 (26.4921, -205.7336) -> (26.4921, -206.0522)
  line L46 (26.4921, -206.0522) -> (25.7832, -206.0522)
  line L47 (25.7832, -206.0522) -> (25.7832, -207.1415)
  spline S62 degree 2 poles (25.7832, -207.1415) (25.7832, -207.3144) (25.7956, -207.5046) (25.8376, -207.5861) knots 0 0 0 1 2 2 2
  spline S63 degree 2 poles (25.8376, -207.5861) (25.8722, -207.6577) (26.0278, -207.7294) (26.1612, -207.7294) knots 0 0 0 1 2 2 2
  spline S64 degree 2 poles (26.1612, -207.7294) (26.255, -207.7294) (26.4304, -207.6725) (26.4699, -207.6553) knots 0 0 0 1 2 2 2
  line L48 (26.4699, -207.6553) -> (26.4921, -207.6553)
  line L49 (26.4921, -207.6553) -> (26.4921, -208.0011)
  spline S65 degree 2 poles (26.4921, -208.0011) (26.3835, -208.0307) (26.1612, -208.0653) (26.0648, -208.0653) knots 0 0 0 1 2 2 2
  spline S66 degree 2 poles (27.4678, -208.0653) (27.1541, -208.0653) (26.8009, -207.7071) (26.8009, -207.3193) knots 0 0 0 1 2 2 2
  line L50 (26.8009, -207.3193) -> (26.8009, -206.0522)
  line L51 (26.8009, -206.0522) -> (26.5415, -206.0522)
  line L52 (26.5415, -206.0522) -> (26.5415, -205.7336)
  line L53 (26.5415, -205.7336) -> (26.8009, -205.7336)
  line L54 (26.8009, -205.7336) -> (26.8009, -205.0766)
  line L55 (26.8009, -205.0766) -> (27.1862, -205.0766)
  line L56 (27.1862, -205.0766) -> (27.1862, -205.7336)
  line L57 (27.1862, -205.7336) -> (27.8951, -205.7336)
  line L58 (27.8951, -205.7336) -> (27.8951, -206.0522)
  line L59 (27.8951, -206.0522) -> (27.1862, -206.0522)
  line L60 (27.1862, -206.0522) -> (27.1862, -207.1415)
  spline S67 degree 2 poles (27.1862, -207.1415) (27.1862, -207.3144) (27.1986, -207.5046) (27.2406, -207.5861) knots 0 0 0 1 2 2 2
  spline S68 degree 2 poles (27.2406, -207.5861) (27.2751, -207.6577) (27.4307, -207.7294) (27.5641, -207.7294) knots 0 0 0 1 2 2 2
  spline S69 degree 2 poles (27.5641, -207.7294) (27.658, -207.7294) (27.8334, -207.6725) (27.8729, -207.6553) knots 0 0 0 1 2 2 2
  line L61 (27.8729, -207.6553) -> (27.8951, -207.6553)
  line L62 (27.8951, -207.6553) -> (27.8951, -208.0011)
  spline S70 degree 2 poles (27.8951, -208.0011) (27.7864, -208.0307) (27.5641, -208.0653) (27.4678, -208.0653) knots 0 0 0 1 2 2 2
  spline S71 degree 2 poles (30.0588, -206.8772) (30.0588, -207.4552) (29.5031, -208.085) (29.0387, -208.085) knots 0 0 0 1 2 2 2
  spline S72 degree 2 poles (29.0387, -208.085) (28.562, -208.085) (28.0161, -207.4354) (28.0161, -206.8772) knots 0 0 0 1 2 2 2
  spline S73 degree 2 poles (28.0161, -206.8772) (28.0161, -206.3042) (28.5793, -205.6694) (29.0387, -205.6694) knots 0 0 0 1 2 2 2
  spline S74 degree 2 poles (29.0387, -205.6694) (29.5031, -205.6694) (30.0588, -206.3017) (30.0588, -206.8772) knots 0 0 0 1 2 2 2
  spline S75 degree 2 poles (29.6612, -206.8772) (29.6612, -206.4326) (29.3376, -206.0003) (29.0387, -206.0003) knots 0 0 0 1 2 2 2
  spline S76 degree 2 poles (29.0387, -206.0003) (28.7399, -206.0003) (28.4138, -206.4326) (28.4138, -206.8772) knots 0 0 0 1 2 2 2
  spline S77 degree 2 poles (28.4138, -206.8772) (28.4138, -207.3095) (28.7399, -207.7541) (29.0387, -207.7541) knots 0 0 0 1 2 2 2
  spline S78 degree 2 poles (29.0387, -207.7541) (29.3351, -207.7541) (29.6612, -207.3169) (29.6612, -206.8772) knots 0 0 0 1 2 2 2
  line L63 (33.0476, -208.0208) -> (33.0476, -206.6969)
  spline S79 degree 2 poles (33.0476, -206.6969) (33.0476, -206.5388) (33.0229, -206.2696) (32.9833, -206.1955) knots 0 0 0 1 2 2 2
  spline S80 degree 2 poles (32.9833, -206.1955) (32.9438, -206.114) (32.7931, -206.0349) (32.6622, -206.0349) knots 0 0 0 1 2 2 2
  spline S81 degree 2 poles (32.6622, -206.0349) (32.5437, -206.0349) (32.272, -206.1807) (32.1287, -206.319) knots 0 0 0 1 2 2 2
  spline S82 degree 2 poles (32.1287, -206.319) (32.1312, -206.3536) (32.1361, -206.4499) (32.1361, -206.5141) knots 0 0 0 1 2 2 2
  line L64 (32.1361, -206.5141) -> (32.1361, -208.0208)
  line L65 (32.1361, -208.0208) -> (31.7508, -208.0208)
  line L66 (31.7508, -208.0208) -> (31.7508, -206.6969)
  spline S83 degree 2 poles (31.7508, -206.6969) (31.7508, -206.5388) (31.7261, -206.2696) (31.6866, -206.1955) knots 0 0 0 1 2 2 2
  spline S84 degree 2 poles (31.6866, -206.1955) (31.6471, -206.114) (31.4964, -206.0349) (31.3655, -206.0349) knots 0 0 0 1 2 2 2
  spline S85 degree 2 poles (31.3655, -206.0349) (31.242, -206.0349) (30.9678, -206.1905) (30.8394, -206.3116) knots 0 0 0 1 2 2 2
  line L67 (30.8394, -206.3116) -> (30.8394, -208.0208)
  line L68 (30.8394, -208.0208) -> (30.454, -208.0208)
  line L69 (30.454, -208.0208) -> (30.454, -205.7336)
  line L70 (30.454, -205.7336) -> (30.8394, -205.7336)
  line L71 (30.8394, -205.7336) -> (30.8394, -205.9855)
  spline S86 degree 2 poles (30.8394, -205.9855) (30.99, -205.8349) (31.2864, -205.6694) (31.4643, -205.6694) knots 0 0 0 1 2 2 2
  spline S87 degree 2 poles (31.4643, -205.6694) (31.6668, -205.6694) (31.9805, -205.8546) (32.062, -206.0646) knots 0 0 0 1 2 2 2
  spline S88 degree 2 poles (32.062, -206.0646) (32.2374, -205.8694) (32.5684, -205.6694) (32.761, -205.6694) knots 0 0 0 1 2 2 2
  spline S89 degree 2 poles (32.761, -205.6694) (32.9092, -205.6694) (33.1513, -205.7608) (33.2402, -205.8645) knots 0 0 0 1 2 2 2
  spline S90 degree 2 poles (33.2402, -205.8645) (33.3316, -205.9682) (33.4329, -206.2795) (33.4329, -206.5141) knots 0 0 0 1 2 2 2
  line L72 (33.4329, -206.5141) -> (33.4329, -208.0208)
  line L73 (33.4329, -208.0208) -> (33.0476, -208.0208)
  spline S91 degree 2 poles (24.8446, -212.1031) (24.8446, -212.3304) (24.6717, -212.6787) (24.5285, -212.7923) knots 0 0 0 1 2 2 2
  spline S92 degree 2 poles (24.5285, -212.7923) (24.3556, -212.9257) (23.9628, -213.0393) (23.6516, -213.0393) knots 0 0 0 1 2 2 2
  line L74 (23.6516, -213.0393) -> (22.7772, -213.0393)
  line L75 (22.7772, -213.0393) -> (22.7772, -209.9913)
  line L76 (22.7772, -209.9913) -> (23.5849, -209.9913)
  spline S93 degree 2 poles (23.5849, -209.9913) (23.911, -209.9913) (24.237, -210.0333) (24.3852, -210.1148) knots 0 0 0 1 2 2 2
  spline S94 degree 2 poles (24.3852, -210.1148) (24.5507, -210.2012) (24.7014, -210.4853) (24.7014, -210.6779) knots 0 0 0 1 2 2 2
  spline S95 degree 2 poles (24.7014, -210.6779) (24.7014, -210.8928) (24.4741, -211.2337) (24.2741, -211.33) knots 0 0 0 1 2 2 2
  line L77 (24.2741, -211.33) -> (24.2741, -211.3448)
  spline S96 degree 2 poles (24.2741, -211.3448) (24.5458, -211.4189) (24.8446, -211.8117) (24.8446, -212.1031) knots 0 0 0 1 2 2 2
  spline S97 degree 2 poles (24.4223, -212.1204) (24.4223, -211.9475) (24.3235, -211.7252) (24.1753, -211.6462) knots 0 0 0 1 2 2 2
  spline S98 degree 2 poles (24.1753, -211.6462) (24.0789, -211.5968) (23.8517, -211.5671) (23.6417, -211.5671) knots 0 0 0 1 2 2 2
  line L78 (23.6417, -211.5671) -> (23.1823, -211.5671)
  line L79 (23.1823, -211.5671) -> (23.1823, -212.6935)
  line L80 (23.1823, -212.6935) -> (23.5108, -212.6935)
  spline S99 degree 2 poles (23.5108, -212.6935) (23.7776, -212.6935) (24.0839, -212.6441) (24.2024, -212.565) knots 0 0 0 1 2 2 2
  spline S100 degree 2 poles (24.2024, -212.565) (24.3161, -212.4835) (24.4223, -212.281) (24.4223, -212.1204) knots 0 0 0 1 2 2 2
  spline S101 degree 2 poles (24.279, -210.7347) (24.279, -210.6261) (24.2049, -210.463) (24.1234, -210.4161) knots 0 0 0 1 2 2 2
  spline S102 degree 2 poles (24.1234, -210.4161) (24.0246, -210.3618) (23.785, -210.3371) (23.5701, -210.3371) knots 0 0 0 1 2 2 2
  line L81 (23.5701, -210.3371) -> (23.1823, -210.3371)
  line L82 (23.1823, -210.3371) -> (23.1823, -211.2288)
  line L83 (23.1823, -211.2288) -> (23.6417, -211.2288)
  spline S103 degree 2 poles (23.6417, -211.2288) (23.8319, -211.2288) (24.0122, -211.1892) (24.1086, -211.1275) knots 0 0 0 1 2 2 2
  spline S104 degree 2 poles (24.1086, -211.1275) (24.2024, -211.0682) (24.279, -210.878) (24.279, -210.7347) knots 0 0 0 1 2 2 2
  spline S105 degree 2 poles (27.0973, -211.8957) (27.0973, -212.4736) (26.5415, -213.1035) (26.0772, -213.1035) knots 0 0 0 1 2 2 2
  spline S106 degree 2 poles (26.0772, -213.1035) (25.6005, -213.1035) (25.0546, -212.4539) (25.0546, -211.8957) knots 0 0 0 1 2 2 2
  spline S107 degree 2 poles (25.0546, -211.8957) (25.0546, -211.3226) (25.6178, -210.6878) (26.0772, -210.6878) knots 0 0 0 1 2 2 2
  spline S108 degree 2 poles (26.0772, -210.6878) (26.5415, -210.6878) (27.0973, -211.3201) (27.0973, -211.8957) knots 0 0 0 1 2 2 2
  spline S109 degree 2 poles (26.6996, -211.8957) (26.6996, -211.4511) (26.376, -211.0188) (26.0772, -211.0188) knots 0 0 0 1 2 2 2
  spline S110 degree 2 poles (26.0772, -211.0188) (25.7783, -211.0188) (25.4523, -211.4511) (25.4523, -211.8957) knots 0 0 0 1 2 2 2
  spline S111 degree 2 poles (25.4523, -211.8957) (25.4523, -212.3279) (25.7783, -212.7725) (26.0772, -212.7725) knots 0 0 0 1 2 2 2
  spline S112 degree 2 poles (26.0772, -212.7725) (26.3736, -212.7725) (26.6996, -212.3353) (26.6996, -211.8957) knots 0 0 0 1 2 2 2
  line L84 (29.2684, -213.0393) -> (28.7967, -213.0393)
  line L85 (28.7967, -213.0393) -> (28.2409, -212.1797)
  line L86 (28.2409, -212.1797) -> (27.6703, -213.0393)
  line L87 (27.6703, -213.0393) -> (27.2331, -213.0393)
  line L88 (27.2331, -213.0393) -> (28.026, -211.9055)
  line L89 (28.026, -211.9055) -> (27.2406, -210.752)
  line L90 (27.2406, -210.752) -> (27.7123, -210.752)
  line L91 (27.7123, -210.752) -> (28.2656, -211.6042)
  line L92 (28.2656, -211.6042) -> (28.8312, -210.752)
  line L93 (28.8312, -210.752) -> (29.2684, -210.752)
  line L94 (29.2684, -210.752) -> (28.4805, -211.8808)
  line L95 (28.4805, -211.8808) -> (29.2684, -213.0393)
  spline S113 degree 2 poles (30.333, -210.2803) (30.2219, -210.2803) (30.002, -210.3346) (29.8958, -210.3766) knots 0 0 0 1 2 2 2
  spline S114 degree 2 poles (29.8958, -210.3766) (29.797, -210.4186) (29.6513, -210.5075) (29.5945, -210.547) knots 0 0 0 1 2 2 2
  line L96 (29.5945, -210.547) -> (29.5698, -210.547)
  line L97 (29.5698, -210.547) -> (29.5698, -210.1148)
  spline S115 degree 2 poles (29.5698, -210.1148) (29.7032, -210.0431) (30.1601, -209.9271) (30.3651, -209.9271) knots 0 0 0 1 2 2 2
  spline S116 degree 2 poles (30.3651, -209.9271) (30.5726, -209.9271) (30.8814, -210.011) (31.0073, -210.1) knots 0 0 0 1 2 2 2
  spline S117 degree 2 poles (31.0073, -210.1) (31.1407, -210.1963) (31.279, -210.4754) (31.279, -210.6631) knots 0 0 0 1 2 2 2
  spline S118 degree 2 poles (31.279, -210.6631) (31.279, -210.9151) (30.948, -211.2954) (30.7159, -211.3448) knots 0 0 0 1 2 2 2
  line L98 (30.7159, -211.3448) -> (30.7159, -211.3745)
  spline S119 degree 2 poles (30.7159, -211.3745) (30.8122, -211.3942) (31.032, -211.4832) (31.1259, -211.5721) knots 0 0 0 1 2 2 2
  spline S120 degree 2 poles (31.1259, -211.5721) (31.2197, -211.6585) (31.3383, -211.9352) (31.3383, -212.1352) knots 0 0 0 1 2 2 2
  spline S121 degree 2 poles (31.3383, -212.1352) (31.3383, -212.3403) (31.1975, -212.6885) (31.0691, -212.8219) knots 0 0 0 1 2 2 2
  spline S122 degree 2 poles (31.0691, -212.8219) (30.9357, -212.9602) (30.5578, -213.1035) (30.3182, -213.1035) knots 0 0 0 1 2 2 2
  spline S123 degree 2 poles (30.3182, -213.1035) (30.0885, -213.1035) (29.6389, -212.9923) (29.4858, -212.9158) knots 0 0 0 1 2 2 2
  line L99 (29.4858, -212.9158) -> (29.4858, -212.4835)
  line L100 (29.4858, -212.4835) -> (29.5154, -212.4835)
  spline S124 degree 2 poles (29.5154, -212.4835) (29.6439, -212.5774) (30.0786, -212.7503) (30.2935, -212.7503) knots 0 0 0 1 2 2 2
  spline S125 degree 2 poles (30.2935, -212.7503) (30.4195, -212.7503) (30.6714, -212.6712) (30.7554, -212.5799) knots 0 0 0 1 2 2 2
  spline S126 degree 2 poles (30.7554, -212.5799) (30.8369, -212.4885) (30.9233, -212.2711) (30.9233, -212.1056) knots 0 0 0 1 2 2 2
  spline S127 degree 2 poles (30.9233, -212.1056) (30.9233, -211.9401) (30.827, -211.7252) (30.7406, -211.6635) knots 0 0 0 1 2 2 2
  spline S128 degree 2 poles (30.7406, -211.6635) (30.6541, -211.6017) (30.4195, -211.5548) (30.2811, -211.5548) knots 0 0 0 1 2 2 2
  line L101 (30.2811, -211.5548) -> (30.1082, -211.5548)
  line L102 (30.1082, -211.5548) -> (30.1082, -211.2164)
  line L103 (30.1082, -211.2164) -> (30.2441, -211.2164)
  spline S129 degree 2 poles (30.2441, -211.2164) (30.5183, -211.2164) (30.8641, -210.9546) (30.8641, -210.7051) knots 0 0 0 1 2 2 2
  spline S130 degree 2 poles (30.8641, -210.7051) (30.8641, -210.589) (30.7751, -210.4235) (30.7035, -210.3741) knots 0 0 0 1 2 2 2
  spline S131 degree 2 poles (30.7035, -210.3741) (30.6269, -210.3223) (30.4392, -210.2803) (30.333, -210.2803) knots 0 0 0 1 2 2 2
  spline S132 degree 2 poles (19.5625, -217.0697) (19.5625, -217.3044) (19.4069, -217.702) (19.276, -217.8354) knots 0 0 0 1 2 2 2
  spline S133 degree 2 poles (19.276, -217.8354) (19.1401, -217.9762) (18.7993, -218.1219) (18.5943, -218.1219) knots 0 0 0 1 2 2 2
  spline S134 degree 2 poles (18.5943, -218.1219) (18.3893, -218.1219) (18.0509, -217.9836) (17.9224, -217.8453) knots 0 0 0 1 2 2 2
  spline S135 degree 2 poles (17.9224, -217.8453) (17.7643, -217.6798) (17.5865, -217.1241) (17.5865, -216.719) knots 0 0 0 1 2 2 2
  spline S136 degree 2 poles (17.5865, -216.719) (17.5865, -216.3213) (17.7495, -215.6816) (17.9199, -215.4444) knots 0 0 0 1 2 2 2
  spline S137 degree 2 poles (17.9199, -215.4444) (18.0854, -215.2123) (18.6091, -214.9529) (18.9524, -214.9529) knots 0 0 0 1 2 2 2
  spline S138 degree 2 poles (18.9524, -214.9529) (19.0537, -214.9529) (19.2315, -214.9727) (19.2982, -214.9949) knots 0 0 0 1 2 2 2
  line L104 (19.2982, -214.9949) -> (19.2982, -215.3876)
  line L105 (19.2982, -215.3876) -> (19.2809, -215.3876)
  spline S139 degree 2 poles (19.2809, -215.3876) (19.2241, -215.358) (19.0166, -215.3061) (18.8981, -215.3061) knots 0 0 0 1 2 2 2
  spline S140 degree 2 poles (18.8981, -215.3061) (18.5177, -215.3061) (18.0509, -215.8199) (18.0064, -216.3238) knots 0 0 0 1 2 2 2
  spline S141 degree 2 poles (18.0064, -216.3238) (18.1521, -216.2225) (18.4584, -216.1114) (18.6412, -216.1114) knots 0 0 0 1 2 2 2
  spline S142 degree 2 poles (18.6412, -216.1114) (18.819, -216.1114) (19.0858, -216.183) (19.2315, -216.2917) knots 0 0 0 1 2 2 2
  spline S143 degree 2 poles (19.2315, -216.2917) (19.3995, -216.4176) (19.5625, -216.8079) (19.5625, -217.0697) knots 0 0 0 1 2 2 2
  spline S144 degree 2 poles (19.1475, -217.087) (19.1475, -216.8993) (19.0487, -216.6449) (18.9401, -216.556) knots 0 0 0 1 2 2 2
  spline S145 degree 2 poles (18.9401, -216.556) (18.8586, -216.4917) (18.656, -216.4497) (18.5498, -216.4497) knots 0 0 0 1 2 2 2
  spline S146 degree 2 poles (18.5498, -216.4497) (18.4065, -216.4497) (18.1373, -216.5362) (18.0064, -216.6177) knots 0 0 0 1 2 2 2
  spline S147 degree 2 poles (18.0064, -216.6177) (18.0039, -216.6622) (17.999, -216.7461) (17.999, -216.8104) knots 0 0 0 1 2 2 2
  spline S148 degree 2 poles (17.999, -216.8104) (17.999, -217.1265) (18.1225, -217.5143) (18.2163, -217.6156) knots 0 0 0 1 2 2 2
  spline S149 degree 2 poles (18.2163, -217.6156) (18.3028, -217.7119) (18.4905, -217.7885) (18.5967, -217.7885) knots 0 0 0 1 2 2 2
  spline S150 degree 2 poles (18.5967, -217.7885) (18.8437, -217.7885) (19.1475, -217.4378) (19.1475, -217.087) knots 0 0 0 1 2 2 2
  line L106 (21.1902, -214.8739) -> (19.9972, -218.7197)
  line L107 (19.9972, -218.7197) -> (19.6514, -218.7197)
  line L108 (19.6514, -218.7197) -> (20.8395, -214.8739)
  line L109 (20.8395, -214.8739) -> (21.1902, -214.8739)
  line L110 (23.2527, -218.0577) -> (21.7658, -218.0577)
  line L111 (21.7658, -218.0577) -> (21.7658, -217.7465)
  line L112 (21.7658, -217.7465) -> (22.319, -217.7465)
  line L113 (22.319, -217.7465) -> (22.319, -215.7038)
  line L114 (22.319, -215.7038) -> (21.7658, -215.7038)
  line L115 (21.7658, -215.7038) -> (21.7658, -215.4247)
  spline S151 degree 2 poles (21.7658, -215.4247) (22.0795, -215.4247) (22.3759, -215.2468) (22.3956, -214.9998) knots 0 0 0 1 2 2 2
  line L116 (22.3956, -214.9998) -> (22.7118, -214.9998)
  line L117 (22.7118, -214.9998) -> (22.7118, -217.7465)
  line L118 (22.7118, -217.7465) -> (23.2527, -217.7465)
  line L119 (23.2527, -217.7465) -> (23.2527, -218.0577)
  line L120 (25.7277, -215.4667) -> (24.4087, -218.0577)
  line L121 (24.4087, -218.0577) -> (23.974, -218.0577)
  line L122 (23.974, -218.0577) -> (25.367, -215.3679)
  line L123 (25.367, -215.3679) -> (23.7936, -215.3679)
  line L124 (23.7936, -215.3679) -> (23.7936, -215.0097)
  line L125 (23.7936, -215.0097) -> (25.7277, -215.0097)
  line L126 (25.7277, -215.0097) -> (25.7277, -215.4667)
  line L127 (27.3678, -214.8739) -> (26.1747, -218.7197)
  line L128 (26.1747, -218.7197) -> (25.8289, -218.7197)
  line L129 (25.8289, -218.7197) -> (27.017, -214.8739)
  line L130 (27.017, -214.8739) -> (27.3678, -214.8739)
  line L131 (29.5834, -218.0577) -> (27.7037, -218.0577)
  line L132 (27.7037, -218.0577) -> (27.7037, -217.6255)
  spline S152 degree 2 poles (27.7037, -217.6255) (27.9062, -217.4353) (28.2668, -217.0821) (28.4397, -216.8919) knots 0 0 0 1 2 2 2
  spline S153 degree 2 poles (28.4397, -216.8919) (28.788, -216.509) (29.0424, -216.0496) (29.0424, -215.8051) knots 0 0 0 1 2 2 2
  spline S154 degree 2 poles (29.0424, -215.8051) (29.0424, -215.6766) (28.9634, -215.484) (28.8918, -215.4222) knots 0 0 0 1 2 2 2
  spline S155 degree 2 poles (28.8918, -215.4222) (28.8201, -215.3605) (28.6324, -215.2987) (28.5188, -215.2987) knots 0 0 0 1 2 2 2
  spline S156 degree 2 poles (28.5188, -215.2987) (28.4101, -215.2987) (28.1878, -215.3531) (28.0865, -215.395) knots 0 0 0 1 2 2 2
  spline S157 degree 2 poles (28.0865, -215.395) (28.0001, -215.4296) (27.8395, -215.5284) (27.7901, -215.563) knots 0 0 0 1 2 2 2
  line L133 (27.7901, -215.563) -> (27.7679, -215.563)
  line L134 (27.7679, -215.563) -> (27.7679, -215.1283)
  spline S158 degree 2 poles (27.7679, -215.1283) (27.8939, -215.0665) (28.3459, -214.9455) (28.5484, -214.9455) knots 0 0 0 1 2 2 2
  spline S159 degree 2 poles (28.5484, -214.9455) (28.9757, -214.9455) (29.4574, -215.3975) (29.4574, -215.7828) knots 0 0 0 1 2 2 2
  spline S160 degree 2 poles (29.4574, -215.7828) (29.4574, -215.9632) (29.3734, -216.2645) (29.2993, -216.3929) knots 0 0 0 1 2 2 2
  spline S161 degree 2 poles (29.2993, -216.3929) (29.2252, -216.5263) (29.0103, -216.7881) (28.8918, -216.9141) knots 0 0 0 1 2 2 2
  spline S162 degree 2 poles (28.8918, -216.9141) (28.6991, -217.1241) (28.2273, -217.5736) (28.0865, -217.7045) knots 0 0 0 1 2 2 2
  line L135 (28.0865, -217.7045) -> (29.5834, -217.7045)
  line L136 (29.5834, -217.7045) -> (29.5834, -218.0577)
  spline S163 degree 2 poles (31.8879, -216.5337) (31.8879, -217.3538) (31.4112, -218.1219) (30.9147, -218.1219) knots 0 0 0 1 2 2 2
  spline S164 degree 2 poles (30.9147, -218.1219) (30.4108, -218.1219) (29.939, -217.339) (29.939, -216.5362) knots 0 0 0 1 2 2 2
  spline S165 degree 2 poles (29.939, -216.5362) (29.939, -215.7112) (30.4158, -214.948) (30.9147, -214.948) knots 0 0 0 1 2 2 2
  spline S166 degree 2 poles (30.9147, -214.948) (31.4161, -214.948) (31.8879, -215.7384) (31.8879, -216.5337) knots 0 0 0 1 2 2 2
  spline S167 degree 2 poles (31.3642, -217.4625) (31.4235, -217.3118) (31.4729, -216.8474) (31.4729, -216.5337) knots 0 0 0 1 2 2 2
  spline S168 degree 2 poles (31.4729, -216.5337) (31.4729, -216.22) (31.4235, -215.7581) (31.3618, -215.6025) knots 0 0 0 1 2 2 2
  spline S169 degree 2 poles (31.3618, -215.6025) (31.3, -215.4469) (31.0851, -215.2864) (30.9147, -215.2864) knots 0 0 0 1 2 2 2
  spline S170 degree 2 poles (30.9147, -215.2864) (30.7443, -215.2864) (30.5244, -215.4469) (30.4602, -215.6075) knots 0 0 0 1 2 2 2
  spline S171 degree 2 poles (30.4602, -215.6075) (30.3985, -215.7631) (30.354, -216.2373) (30.354, -216.5362) knots 0 0 0 1 2 2 2
  spline S172 degree 2 poles (30.354, -216.5362) (30.354, -216.8573) (30.3935, -217.2871) (30.4577, -217.455) knots 0 0 0 1 2 2 2
  spline S173 degree 2 poles (30.4577, -217.455) (30.517, -217.6131) (30.7369, -217.7836) (30.9147, -217.7836) knots 0 0 0 1 2 2 2
  spline S174 degree 2 poles (30.9147, -217.7836) (31.0827, -217.7836) (31.3025, -217.623) (31.3642, -217.4625) knots 0 0 0 1 2 2 2
  line L137 (34.1578, -218.0577) -> (32.2782, -218.0577)
  line L138 (32.2782, -218.0577) -> (32.2782, -217.6255)
  spline S175 degree 2 poles (32.2782, -217.6255) (32.4807, -217.4353) (32.8413, -217.0821) (33.0142, -216.8919) knots 0 0 0 1 2 2 2